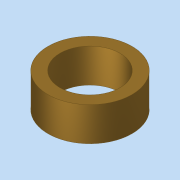
# Autodesk Inventor part: BrassMountInserts
Saved by Autodesk Inventor 2017 (Build 210142000, 142)
## iProperties
Created: 2018-04-09
Part Number: BrassMountInserts
Material: Brass, Soft Yellow
Document SubType Name: Modeling
Designer: Derek Wider
Density: 8.47 g/cm^3
Appearance: Brass - Satin
Author: Derek Wider
Autodesk Inventor part; units mm, degrees
ref_plane "YZ Plane" through (0, 0, 0) normal (1, 0, 0) x (0, 1, 0)
ref_plane "XZ Plane" through (0, 0, 0) normal (0, 1, 0) x (-1, 0, 0)
ref_plane "XY Plane" through (0, 0, 0) normal (0, 0, 1) x (1, 0, 0)
sketch "Sketch1" plane through (0, 0, 0) normal (0, 1, 0) x (-1, 0, 0)
  circle A0 centre (0, 0) radius 1.778
  circle A1 centre (0, 0) radius 2.4892
  dimension "d0" = 3.556
  dimension "d1" = 4.9784
  constraints: 2 centre point, 2 coincident
  measures "d0" diameter of A0
  measures "d1" diameter of A1
extrude "Extrusion1" add sketch "Sketch1" along normal blind 2.0066
body "Solid1"
